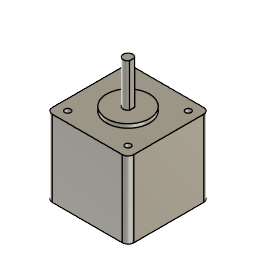
Servo from 3d printer (Autodesk Fusion 360 design; units mm, degrees)
Autodesk Fusion 360 part; units mm, degrees
box "BoxPrimitive1" add length 42 width 42 height 39.3 placed x (0, -1, 0) y (1, 0, 0) z (0, 0, 1) at (0, 0, 0)
sketch "Sketch2" plane through (0, 0, 39.3) normal (0, 0, 1) x (-1, 0, 0)
  line L0 (0, 42) -> (-42, 42)
  line L1 (-42, 42) -> (-42, 0)
  line L2 (-42, 0) -> (0, 0)
  line L3 (0, 0) -> (0, 42)
  circle A0 centre (-21, 21) radius 11
  line L4 (-23.1, 22.3565) -> (-23.1, 19.6435)
  arc A1 (-23.1, 19.6435) -> (-23.1, 22.3565) centre (-21, 21) ccw
  circle A2 centre (-36.5, 36.5) radius 1.5
  circle A3 centre (-5.5, 36.5) radius 1.5
  line L5 (-5.5, 36.5) -> (-36.5, 36.5) construction
  line L6 (-36.5, 36.5) -> (-36.5, 5.5) construction
  circle A4 centre (-36.5, 5.5) radius 1.5
  circle A5 centre (-5.5, 5.5) radius 1.5
  point P0 (-21, 0)
  point P1 (0, 21)
  point P2 (-21, 36.5)
  point P3 (-21, 42)
  point P4 (-36.5, 21)
  point P5 (-42, 21)
  dimension "d8" = 22
  dimension "d11" = 5
  dimension "d14" = 2.1
  dimension "d17" = 3
  dimension "d20" = 3
  dimension "d21" = 31
  dimension "d22" = 31
  dimension "d23" = 3
  dimension "d24" = 3
  constraint midpoint L2 P0
  constraint vertical A0.centre P0
  constraint midpoint L3 P1
  constraint horizontal A0.centre P1
  constraint concentric A0 A1
  constraint vertical L4
  constraint coincident A3.centre L5.start
  constraint coincident A2.centre L5.end
  constraint midpoint L5 P2
  constraint midpoint L0 P3
  constraint vertical P2 P3
  constraint horizontal L5
  constraint perpendicular L5 L6
  constraint coincident L6.end A4.centre
  constraint midpoint L6 P4
  constraint midpoint L1 P5
  constraint horizontal P4 P5
  constraint vertical A3.centre A5.centre
  constraint horizontal L6.end A5.centre
  measures "d8" diameter of A0
  measures "d11" diameter of A1
  measures "d14" distance of A0.centre L4
  measures "d17" diameter of A2
  measures "d20" diameter of A3
  measures "d21" distance of A3.centre A2.centre
  measures "d22" distance of A2.centre L6.end
  measures "d23" diameter of A4
  measures "d24" diameter of A5
extrude "Extrude2" add sketch "Sketch2" along normal blind 24 contours L4 A1
extrude "Extrude1" add sketch "Sketch2" along normal blind 2 contours A0 | L4 A1
fillet "Fillet1" radius 3 4 edges at (0, 0, 19.65) (0, -42, 19.65) (42, -42, 19.65) (42, 0, 19.65)
extrude "Extrude3" cut sketch "Sketch2" against normal blind 40 contours A2 | A3 | A4 | A5
